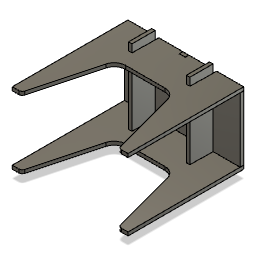
Mesa (Autodesk Fusion 360 design; units mm, degrees)
Autodesk Fusion 360 part; units mm, degrees
sketch "Boceto1" plane through (0, 0, 0) normal (0, 1, 0) x (1, 0, 0)
  line L0 (94.3029, 0) -> (100, 0)
  line L1 (100, 0) -> (100, 100)
  line L2 (100, 100) -> (0, 100)
  line L3 (0, 100) -> (0, 0)
  line L4 (0, 0) -> (5.698, 0)
  line L5 (0, 100) -> (0, 65)
  line L6 (33.09, 65) -> (66.9346, 65)
  line L7 (8.5958, 2.2235) -> (23.4307, 57.5882)
  line L8 (8, 0) -> (75.1863, 0) construction
  line L9 (100, 0) -> (92, 0)
  line L10 (75, 65) -> (74.611, 65)
  line L11 (91.4048, 2.2247) -> (76.5949, 57.5843)
  arc A0 (91.4048, 2.2247) -> (94.3029, 0) centre (94.3029, 3) ccw
  arc A1 (5.698, 0) -> (8.5958, 2.2235) centre (5.698, 3) ccw
  arc A2 (33.09, 65) -> (23.4307, 57.5882) centre (33.09, 55) ccw
  arc A3 (76.5949, 57.5843) -> (66.9346, 65) centre (66.9346, 55) ccw
  line L12 (0, 100) -> (25, 100)
  line L13 (25, 100) -> (25, 60.8781) construction
  line L14 (100, 100) -> (75, 100)
  line L15 (75, 100) -> (75, 60.9118) construction
  line L16 (23.4, 100) -> (23.4, 87)
  line L17 (23.4, 87) -> (26.6, 87)
  line L18 (26.6, 100) -> (26.6, 87)
  line L19 (73.4, 100) -> (73.4, 87)
  line L20 (73.4, 87) -> (76.6, 87)
  line L21 (76.6, 100) -> (76.6, 87)
  dimension "d1" = 100
  dimension "d2" = 100
  dimension "d3" = 100
  dimension "d4" = 8
  dimension "d5" = 35
  dimension "d6" = 75
  dimension "d7" = 8
  dimension "d9" = 3
  dimension "d10" = 3
  dimension "d11" = 10
  dimension "d12" = 10
  dimension "d16" = 25
  dimension "d17" = 25
  dimension "d18" = 13
  dimension "d19" = 3.2
  dimension "d20" = 13
  dimension "d21" = 3.2
  constraint coincident L3.end L4.start
  constraint horizontal L0
  constraint perpendicular L0 L1
  constraint perpendicular L1 L2
  constraint perpendicular L3 L4
  constraint perpendicular L2 L5
  constraint perpendicular L1 L6
  constraint horizontal L8
  constraint perpendicular L1 L9
  constraint coincident L6 L10.end
  constraint coincident L3.end L0
  constraint coincident L9.end L11
  constraint tangent L0 A0
  constraint tangent L11 A0
  constraint coincident L8.start L4
  constraint coincident L8.start L7
  constraint tangent L4 A1
  constraint tangent L7 A1
  constraint coincident L5.end L6
  constraint tangent L7 A2
  constraint tangent L6 A2
  constraint coincident L10.end L11
  constraint tangent L11 A3
  constraint tangent L6 A3
  constraint perpendicular L3 L12
  constraint coincident A2 L13.end
  constraint perpendicular L12 L13
  constraint perpendicular L1 L14
  constraint coincident A3 L15.end
  constraint perpendicular L10 L15
  constraint coincident L2 L16.start
  constraint perpendicular L2 L16
  constraint perpendicular L16 L17
  constraint symmetric L13 L16.start L18.start
  constraint symmetric L13 L16.end L17.end
  constraint coincident L2 L19.start
  constraint perpendicular L2 L19
  constraint perpendicular L19 L20
  constraint symmetric L15 L19.start L21.start
  constraint symmetric L15 L19.end L20.end
  constraint coincident L15 L10.start
  measures "d1" distance of L3.end L0.end
  measures "d2" distance of L0.end L1.end
  measures "d3" distance of L1.end L2.end
  measures "d4" distance of L3.end L8.start
  measures "d5" distance of L2.end L5.end
  measures "d6" angle of L7 L8
  measures "d7" distance of L0.end L9.end
  measures "d9" radius of A0
  measures "d10" radius of A1
  measures "d11" radius of A2
  measures "d12" radius of A3
  measures "d16" distance of L2.end L12.end
  measures "d17" distance of L1.end L14.end
  measures "d18" distance of L16.start L16.end
  measures "d19" distance of L16.start L18.start
  measures "d20" distance of L19.start L19.end
  measures "d21" distance of L19.start L21.start
extrude "Extruir1" add sketch "Boceto1" along normal mid plane 3 contours L0 L1 L2 L3 L4 L5 L6 L7 L9 L11 A0 A1 A2 A3 L12 L14 L16 L17 L18 L19 L20 L21 makes body 1
copy_body "CopiarPegarCuerpos1" bodies 1 makes body 2
copy_body "CopiarPegarCuerpos2" bodies 1 makes body 3
move_body "Desplazar1" bodies 3 to x (1, 0, 0) y (0, 1, 0) z (0, 0, 1) at (0, 55.5, 0)
sketch "Boceto2" plane through (100, 0, 0) normal (1, 0, 0) x (0, 0, -1)
  line L0 (100, 54) -> (100, 57)
  line L1 (100, 57) -> (0, 57)
  line L2 (0, 57) -> (0, 54)
  line L3 (0, 54) -> (100, 54)
  line L4 (130, 0) -> (130, 55.5)
  line L5 (130, 55.5) -> (130, 65.5)
  line L6 (130, 0) -> (130, -10)
  line L7 (130, 0) -> (140, 0)
  line L8 (140, 0) -> (140, -3.2)
  line L9 (140, -3.2) -> (130, -3.2)
  line L10 (140, 55.5313) -> (140.0141, 58.7)
  line L11 (140.0141, 58.7) -> (130, 58.7)
  line L12 (130, -10) -> (130, -1.6)
  line L13 (140, -1.5133) -> (150, -1.5133) construction
  line L14 (130, 65.5) -> (130, 57.1)
  line L15 (130, 57.1) -> (150, 57.1) construction
  line L16 (140.0141, 55.5) -> (130, 55.5)
  line L17 (140.0141, 55.5) -> (140.0141, 58.7)
  line L18 (130, 65.5) -> (150, 65.5)
  line L19 (130, -10) -> (150, -10)
  line L20 (150, -10) -> (150, 65.5)
  dimension "d24" = 55.5
  dimension "d25" = 10
  dimension "d26" = 10
  dimension "d27" = 10
  dimension "d28" = 8.4
  dimension "d29" = 8.4
  dimension "d30" = 3.2
  dimension "d31" = 3.2
  dimension "d32" = 20
  dimension "d33" = 20
  dimension "d34" = 10
  constraint vertical L4
  constraint parallel L4 L5
  constraint parallel L4 L6
  constraint perpendicular L6 L7
  constraint perpendicular L7 L8
  constraint coincident L6 L9.end
  constraint perpendicular L6 L9
  constraint coincident L5 L11.end
  constraint horizontal L11
  constraint parallel L6 L12
  constraint perpendicular L6 L13
  constraint perpendicular L14 L15
  constraint symmetric L10.end L15 L16.start
  constraint symmetric L11.end L15 L4.end
  constraint perpendicular L11 L17
  constraint perpendicular L5 L18
  constraint perpendicular L6 L19
  constraint coincident L20 L15.end
  constraint coincident L8 L13.start
  constraint coincident L20 L13.end
  measures "d24" distance of L4.start L4.end
  measures "d25" distance of L4.end L5.end
  measures "d26" distance of L4.start L6.end
  measures "d27" distance of L4.end L10.start
  measures "d28" distance of L6.end L12.end
  measures "d29" distance of L5.end L14.end
  measures "d30" distance of L11 L16
  measures "d31" distance of L7 L9
  measures "d32" distance of L5.end L18.end
  measures "d33" distance of L6.end L19.end
  measures "d34" distance of L8.end L9.end
extrude "Extruir2" add sketch "Boceto2" along normal mid plane 3 separate body contours L4 L5 L6 L7 L8 L9 L11 L12 L14 L16 L17 L18 L19 L20 makes body 4
copy_body "CopiarPegarCuerpos3" bodies 4 makes body 5
move_body "Desplazar2" bodies 5 to x (1, 0, 0) y (0, 1, 0) z (0, 0, 1) at (-50, 0, 0)
move_body "Desplazar3" bodies 4 to x (1, 0, 0) y (0, 1, 0) z (0, 0, 1) at (-25, -1.6, 53.0141)
move_body "Desplazar4" bodies 5 to x (1, 0, 0) y (0, 1, 0) z (0, 0, 1) at (-25, -1.6, 53.0141)
move_body "Desplazar5" bodies 1 2 to x (1, 0, 0) y (0, 1, 0) z (0, 0, 1) at (0, -3.2, 0)
sketch "Boceto3" plane through (0, 57, 0) normal (0, 1, 0) x (-1, 0, 0)
  line L0 (-100, 0) -> (-100, -100)
  line L1 (-100, -100) -> (-76.6, -100)
  line L2 (-76.6, -100) -> (-76.6, -87)
  line L3 (-76.6, -87) -> (-73.4, -87)
  line L4 (-73.4, -87) -> (-73.4, -100)
  line L5 (-73.4, -100) -> (-26.6, -100)
  line L6 (-26.6, -100) -> (-26.6, -87)
  line L7 (-26.6, -87) -> (-23.4, -87)
  line L8 (-23.4, -87) -> (-23.4, -100)
  line L9 (-23.4, -100) -> (0, -100)
  line L10 (0, -100) -> (0, 0)
  line L11 (0, 0) -> (-5.698, 0)
  arc A0 (-5.698, 0) -> (-8.5958, -2.2235) centre (-5.698, -3) ccw
  line L12 (-8.5958, -2.2235) -> (-23.4307, -57.5882)
  arc A1 (-33.09, -65) -> (-23.4307, -57.5882) centre (-33.09, -55) ccw
  line L13 (-33.09, -65) -> (-66.9346, -65)
  arc A2 (-76.5949, -57.5843) -> (-66.9346, -65) centre (-66.9346, -55) ccw
  line L14 (-76.5949, -57.5843) -> (-91.4048, -2.2247)
  arc A3 (-91.4048, -2.2247) -> (-94.3029, 0) centre (-94.3029, -3) ccw
  line L15 (-94.3029, 0) -> (-100, 0)
  line L16 (-26.6, -100) -> (-47.4, -100)
  line L17 (-50, -100) -> (-50.0123, -65) construction
  line L18 (-50.99, -100) -> (-50.99, -100.0007)
  line L19 (-47.4, -100) -> (-47.4, -96.9)
  line L20 (-47.4, -96.9) -> (-52.6, -96.9)
  line L21 (-52.6, -100.0018) -> (-52.696, -100)
  line L22 (-47.4022, -96.8982) -> (-47.4022, -96.9)
  line L23 (-52.6, -96.9) -> (-52.6, -100)
  dimension "d45" = 23.4
  dimension "d46" = 3.1
  dimension "d47" = 5.2
  constraint coincident L5.end L6.start
  constraint perpendicular L6 L16
  constraint midpoint L13 L17.end
  constraint coincident L5 L16.end
  constraint perpendicular L5 L19
  constraint perpendicular L19 L20
  constraint symmetric L17 L16.end L21.start
  constraint symmetric L17 L20.end L22.start
  constraint coincident L5 L21.end
  constraint coincident L20 L22.end
  constraint coincident L5 L23.end
  constraint perpendicular L5 L23
  measures "d45" distance of L5.end L17.start
  measures "d46" distance of L16.end L19.end
  measures "d47" distance of L19.end L20.end
extrude "Extruir3" cut sketch "Boceto3" against normal blind 3 contours L5 L19 L20 L23 bodies 3
sketch "Boceto4" plane through (0, -4.7, 0) normal (0, -1, 0) x (1, 0, 0)
  line L0 (100, -100) -> (100, 0)
  line L1 (100, 0) -> (94.3029, 0)
  arc A0 (94.3029, 0) -> (91.4048, -2.2247) centre (94.3029, -3) ccw
  line L2 (91.4048, -2.2247) -> (76.5949, -57.5843)
  arc A1 (66.9346, -65) -> (76.5949, -57.5843) centre (66.9346, -55) ccw
  line L3 (66.9346, -65) -> (33.09, -65)
  arc A2 (23.4307, -57.5882) -> (33.09, -65) centre (33.09, -55) ccw
  line L4 (23.4307, -57.5882) -> (8.5958, -2.2235)
  arc A3 (8.5958, -2.2235) -> (5.698, 0) centre (5.698, -3) ccw
  line L5 (5.698, 0) -> (0, 0)
  line L6 (0, -100) -> (23.4, -100)
  line L7 (23.4, -100) -> (23.4, -87)
  line L8 (23.4, -87) -> (26.6, -87)
  line L9 (26.6, -87) -> (26.6, -100)
  line L10 (26.6, -100) -> (73.4, -100)
  line L11 (73.4, -100) -> (73.4, -87)
  line L12 (73.4, -87) -> (76.6, -87)
  line L13 (76.6, -87) -> (76.6, -100)
  line L14 (76.6, -100) -> (100, -100)
  line L15 (50, -100) -> (50.0123, -65) construction
  line L16 (52.6, -100.0009) -> (52.6, -100)
  line L17 (52.6, -100.0009) -> (47.4, -99.9991)
  line L18 (73.4, -100, -3) -> (26.6, -100, -3)
  line L19 (52.6, -100, 0) -> (52.6, -100, -3)
  line L20 (47.4, -99.9991, 0) -> (47.4, -99.9991, -3)
  line L21 (52.6, -100, -3) -> (47.4, -99.9991, -3)
  line L22 (52.6, -100) -> (47.4, -99.9991)
  dimension "d51" = 2.6
  dimension "d52" = 2.6
  dimension "d55" = 3
  constraint midpoint L10 L15.start
  constraint midpoint L3 L15.end
  constraint perpendicular L10 L16
  constraint coincident L10 L16.end
  measures "d51" distance of L15.start L16.start
  measures "d52" distance of L15.start L17.end
  measures "d55" distance of L17.end L22.end
extrude "Extruir4" cut sketch "Boceto4" against normal blind 5.2 contours L19 L20 L21 L22 in plane through (-0.0175, -4.7, -99.9908) normal (0.000175, 0, 1) bodies 1 2
extrude "Extruir5" cut 2 faces at (47.4, -3.7, -99.9994) (50.8667, -3.7, -99.9997) along direction (0.000175, 0, 1) blind 5.2 on bodies 1 bodies 1 2
sketch "Boceto5" plane through (0, 0, 0) normal (0, 0, 1) x (1, 0, 0)
  line L0 (-40, 54, -100) -> (-40, -1.7, -100)
  line L1 (-140, -1.7, -100) -> (-140, 54, -100)
  line L2 (-40, 54, -100) -> (-87.4, 54, -100)
  line L3 (-140, 54, -100) -> (-92.6, 54, -100)
  line L4 (-90, 57, -100) -> (-90, 54, -100) construction
  line L5 (-87.4, 54, -100) -> (-87.4, 57, -100)
  line L6 (-87.4, 57, -100) -> (-92.6, 57, -100)
  line L7 (-92.6, 57, -100) -> (-92.6, 54, -100)
  line L8 (-40, 54, -100) -> (-87.4, 54, -100)
  line L9 (-92.6, 54, -100) -> (-140, 54, -100)
  line L10 (-140, -1.7, -100) -> (-92.6, -1.7, -100)
  line L11 (-90, -1.7, -100) -> (-90, -8, -100)
  line L12 (-90, -8, -100) -> (-90, -1.7, -100) construction
  line L13 (-87.4, -1.7, -100) -> (-87.4, -4.7, -100)
  line L14 (-87.4, -4.7, -100) -> (-92.6, -4.7, -100)
  line L15 (-92.6, -4.7, -100) -> (-92.6, -1.7, -100)
  line L16 (-40, -1.7, -100) -> (-87.4, -1.7, -100)
  dimension "d61" = 55.7
  dimension "d62" = 100
  dimension "d63" = 100
  dimension "d64" = 47.4
  dimension "d65" = 47.4
  dimension "d66" = 3
  dimension "d67" = 5.2
  dimension "d68" = 47.4
  dimension "d69" = 47.4
  dimension "d72" = 3
  dimension "d73" = 5.2
extrude "Extruir6" add sketch "Boceto5" along normal mid plane 3 separate body contours L0 L1 L2 L3 L5 L6 L7 L8 L9 L10 L13 L14 L15 L16 in plane through (0, 0, -100) normal (0, 0, 1) makes body 6
sketch "Boceto6" plane through (0, -4.7, 0) normal (0, -1, 0) x (1, 0, 0)
  line L0 (52.6009, -94.8) -> (52.6, -100)
  line L1 (52.6, -100) -> (73.4, -100)
  line L2 (73.4, -100) -> (73.4, -87)
  line L3 (73.4, -87) -> (76.6, -87)
  line L4 (76.6, -87) -> (76.6, -100)
  line L5 (76.6, -100) -> (100, -100)
  line L6 (100, -100) -> (100, 0)
  line L7 (100, 0) -> (94.3029, 0)
  arc A0 (94.3029, 0) -> (91.4048, -2.2247) centre (94.3029, -3) ccw
  line L8 (91.4048, -2.2247) -> (76.5949, -57.5843)
  arc A1 (66.9346, -65) -> (76.5949, -57.5843) centre (66.9346, -55) ccw
  line L9 (66.9346, -65) -> (33.09, -65)
  arc A2 (23.4307, -57.5882) -> (33.09, -65) centre (33.09, -55) ccw
  line L10 (23.4307, -57.5882) -> (8.5958, -2.2235)
  arc A3 (8.5958, -2.2235) -> (5.698, 0) centre (5.698, -3) ccw
  line L11 (5.698, 0) -> (0, 0)
  line L12 (0, 0) -> (0, -100)
  line L13 (0, -100) -> (23.4, -100)
  line L14 (23.4, -100) -> (23.4, -87)
  line L15 (23.4, -87) -> (26.6, -87)
  line L16 (26.6, -87) -> (26.6, -100)
  line L17 (26.6, -100) -> (47.4, -100)
  line L18 (47.4, -100) -> (47.4009, -94.7991)
  line L19 (47.4009, -94.7991) -> (52.6009, -94.8)
  line L20 (52.6, -100) -> (52.6, -96.9)
  line L21 (52.6, -96.9) -> (47.4005, -96.8991)
  constraint coincident L0.end L1.start
  constraint perpendicular L1 L20
  constraint coincident L18 L21.end
  constraint perpendicular L18 L21
extrude "Extruir7" add sketch "Boceto6" against normal blind 3 contours L0 L18 L19 L20 L21 bodies 1 4 5 2
move_body "Desplazar6" bodies 6 to x (1, 0, 0) y (0, 1, 0) z (0, 0, 1) at (140.0003, 0, 1.5505)
sketch "Boceto7" plane through (0, 0, 0) normal (1, 0, 0) x (0, 0, -1)
equation "MitadespesorMDF = 1.5 mm"
equation "EspesorMDF = 3 mm"
equation "Holgura = 0.1 mm"
equation "d19 = EspesorMDF + Holgura * 2"
equation "d21 = EspesorMDF + Holgura * 2"
equation "d22 = MitadespesorMDF"
equation "d30 = EspesorMDF + Holgura * 2"
equation "d31 = EspesorMDF + Holgura * 2"
equation "d35 = MitadespesorMDF"
equation "d46 = Holgura + 3 mm"
equation "d47 = Holgura * 2 + 5 mm"
equation "d66 = EspesorMDF"
equation "d67 = Holgura * 2 + 5 mm"
equation "d72 = EspesorMDF"
equation "d74 = MitadespesorMDF"
